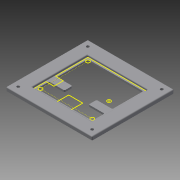
# Autodesk Inventor part: Programming_Jig_Holder
Saved by Autodesk Inventor 2013 (Build 170138000, 138)
## iProperties
Created: 2013-08-23
Part Number: Programming_Jig_Holder
Material: Generic
Document SubType Name: Modeling
Designer: md
Density: 1 g/cm^3
Author: md
Autodesk Inventor part; units mm, degrees
ref_plane "YZ Plane" through (0, 0, 0) normal (1, 0, 0) x (0, 1, 0)
ref_plane "XZ Plane" through (0, 0, 0) normal (0, 1, 0) x (-1, 0, 0)
ref_plane "XY Plane" through (0, 0, 0) normal (0, 0, 1) x (1, 0, 0)
derived "Mockup_Platinen.ipt"
sketch "Umriss_Sensorplatine" plane through (0, 0, 0) normal (0, 0, 1) x (1, 0, 0)
  line L0 (0, 62) -> (67, 62)
  line L1 (67, 62) -> (67, 0)
  line L2 (67, 0) -> (42, 0)
  line L3 (42, 0) -> (42, 14)
  line L4 (42, 14) -> (26, 14)
  line L5 (26, 14) -> (26, 0)
  line L6 (26, 0) -> (0, 0)
  line L7 (0, 14.3) -> (9, 14.3)
  line L8 (9, 14.3) -> (9, 25)
  line L9 (9, 25) -> (0, 25)
  line L10 (0, 0) -> (0, 14.3)
  line L11 (0, 25) -> (0, 62)
  circle A0 centre (63, 4) radius 2
  circle A1 centre (4, 4) radius 2
  circle A2 centre (55, 31) radius 2
  circle A3 centre (4, 58) radius 2
  line L12 (4, 4) -> (63, 4) construction
  line L13 (4, 4) -> (4, 58) construction
sketch "Sketch2" plane through (0, 0, 0) normal (0, 0, 1) x (1, 0, 0)
  line L0 (0, 62) -> (67, 62) projected
  line L1 (0, 25) -> (0, 62) projected
  line L2 (0, 0) -> (0, 14.3) projected
  line L3 (26, 0) -> (0, 0) projected
  line L4 (67, 0) -> (42, 0) projected
  line L5 (67, 62) -> (67, 0) projected
  line L6 (0, 25) -> (0, 14.3)
  line L7 (26, 0) -> (42, 0)
  line L8 (67.6, 62.6) -> (-0.6, 62.6)
  line L9 (-0.6, 62.6) -> (-0.6, 25)
  line L10 (-0.6, 25) -> (-0.6, 14.3)
  line L11 (-0.6, 14.3) -> (-0.6, -0.6)
  line L12 (-0.6, -0.6) -> (26, -0.6)
  line L13 (26, -0.6) -> (42, -0.6)
  line L14 (42, -0.6) -> (67.6, -0.6)
  line L15 (67.6, -0.6) -> (67.6, 62.6)
  line L16 (-15.6, 77.6) -> (82.6, 77.6)
  line L17 (82.6, 77.6) -> (82.6, -15.6)
  line L18 (82.6, -15.6) -> (42, -15.6)
  line L19 (42, -15.6) -> (26, -15.6)
  line L20 (26, -15.6) -> (-15.6, -15.6)
  line L21 (-15.6, -15.6) -> (-15.6, 14.3)
  line L22 (-15.6, 14.3) -> (-15.6, 25)
  line L23 (-15.6, 25) -> (-15.6, 77.6)
  dimension "d1" = 0.6
  dimension "d2" = 15
  constraints: 36 end point, 3 parallel, 3 perpendicular, 14 other
  measures "d1" distance between parallel lines of L8 L0
  measures "d2" distance between parallel lines of L16 L8
extrude "Extrusion1" add sketch "Sketch2" along normal blind 2 contours L16 L17 L18 L19 L20 L21 L22 L23
sketch "Sketch3" plane through (0, 0, 0) normal (0, 0, -1) x (-1, 0, 0)
  line L0 (15.6, 77.6) -> (-82.6, 77.6) projected
  line L1 (-82.6, 77.6) -> (-82.6, -15.6) projected
  line L2 (-82.6, -15.6) -> (15.6, -15.6) projected
  line L3 (15.6, -15.6) -> (15.6, 77.6) projected
  line L4 (0, 62) -> (-67, 62) projected
  line L5 (-67, 62) -> (-67, 0) projected
  line L6 (-67, 0) -> (-42, 0) projected
  line L7 (-26, 0) -> (0, 0) projected
  line L8 (0, 0) -> (0, 14.3) projected
  line L9 (0, 25) -> (0, 62) projected
  line L10 (-65, 60) -> (-2, 60)
  line L11 (-2, 60) -> (-2, 25)
  line L12 (-2, 16) -> (-2, 2)
  line L13 (-2, 2) -> (-65, 2)
  line L14 (0.6, 62.6) -> (0.6, -0.6) projected
  line L15 (-2, 16) -> (-19.4, 16)
  line L16 (-19.4, 16) -> (-19.4, 25)
  line L17 (-65, 16) -> (-47, 16)
  line L18 (-47, 16) -> (-47, 25)
  line L19 (-47, 25) -> (-65, 25)
  line L20 (-65, 2) -> (-65, 16)
  line L21 (-65, 25) -> (-65, 60)
  line L22 (-67.6, 62.6) -> (0.6, 62.6) projected
  line L23 (-2, 25) -> (-19.4, 25)
  dimension "d5" = 2
  dimension "d14" = 35
  dimension "d16" = 44
  dimension "d18" = 2
  dimension "d19" = 20
  dimension "d20" = 20
  dimension "d21" = 2
  constraints: 24 end point, 4 collinear, 2 horizontal, 2 parallel, 2 perpendicular, 1 other
  measures "d5" distance between parallel lines of L4 L10
  measures "d14" distance between parallel lines of L10 L19
  measures "d16" distance between parallel lines of L17 L10
  measures "d18" distance between parallel lines of L5 L21
  measures "d19" distance between parallel lines of L5 L18
  measures "d20" distance between parallel lines of L14 L16
  measures "d21" distance between parallel lines of L7 L13
extrude "Extrusion4" add sketch "Sketch3" along normal blind 2
sketch "Sketch4" plane through (0, 0, 2) normal (0, 0, 1) x (1, 0, 0)
  line L0 (82.6, 77.6) -> (-15.6, 77.6) projected
  line L1 (-15.6, 77.6) -> (-15.6, -15.6) projected
  line L2 (-15.6, -15.6) -> (82.6, -15.6) projected
  line L3 (82.6, -15.6) -> (82.6, 77.6) projected
  line L4 (67.6, 62.6) -> (82.6, 77.6) construction
  line L5 (-15.6, 77.6) -> (-0.6, 62.6) construction
  line L6 (67.6, -0.6) -> (82.6, -15.6) construction
  line L7 (-0.6, -0.6) -> (-15.6, -15.6) construction
  line L8 (-8.6, 70.6) -> (75.6, 70.6) construction
  line L9 (75.6, 70.6) -> (75.6, -8.6) construction
  line L10 (75.6, -8.6) -> (-8.6, -8.6) construction
  line L11 (-8.6, -8.6) -> (-8.6, 70.6) construction
  circle A0 centre (75.6, 70.6) radius 1.6
  circle A1 centre (-8.6, 70.6) radius 1.6
  circle A2 centre (-8.6, -8.6) radius 1.6
  circle A3 centre (75.6, -8.6) radius 1.6
  point P0 (0, 0)
  dimension "d8" = 7
  dimension "d9" = 3.2
  constraints: 16 end point, 4 centre point, 4 coincident, 3 equal radius, 2 perpendicular, 1 parallel, 3 other
  measures "d8" distance between parallel lines of L0 L8
  measures "d9" diameter of A0
extrude "Extrusion3" cut sketch "Sketch4" against normal up to next contours A0 | A1 | A2 | A3
fillet "Fillet1" radius 1 12 edges at (33.5, 77.6, 2) (-15.6, 31, 2) (33.5, -15.6, 2) (82.6, 31, 2) (82.6, 77.6, 0) (82.6, -15.6, 0) (-15.6, -15.6, 0) (-15.6, 77.6, 0) (67.6, 31, 2) (33.5, -0.6, 2) (-0.6, 31, 2) (33.5, 62.6, 2)
fillet "Fillet2" radius 1 8 edges at (67.8929, -0.8929, 1.7071) (67.6, -0.6, 0.5) (-0.6, -0.6, 0.5) (-0.8929, -0.8929, 1.7071) (67.6, 62.6, 0.5) (67.8929, 62.8929, 1.7071) (-0.6, 62.6, 0.5) (-0.8929, 62.8929, 1.7071)
fillet "Fillet3" radius 1 12 edges at (65, 60, -1) (65, 16, -1) (65, 25, -1) (65, 2, -1) (2, 2, -1) (2, 60, -1) (47, 25, -1) (47, 16, -1) (19.4, 16, -1) (19.4, 25, -1) (2, 25, -1) (2, 16, -1)
equation "\"d18\" = d5"
equation "\"d21\" = d5"
body "Solid1"
